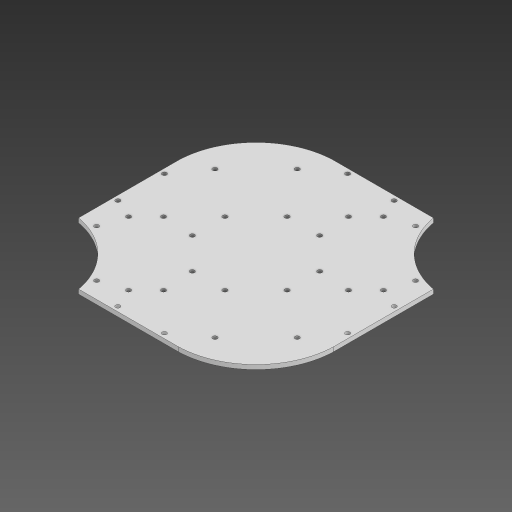
# Autodesk Inventor part: plat
Saved by Autodesk Inventor 2023 (Build 270158000, 158)
## iProperties
Created: 2025-06-24
Part Number: plat
Material: Типовые
Document SubType Name: Modeling
Designer: daa
Density: 1 g/cm^3
Appearance: По умолчанию
Author: daa
Autodesk Inventor part; units mm, degrees
ref_plane "YZ Plane" through (0, 0, 0) normal (1, 0, 0) x (0, 1, 0)
ref_plane "XZ Plane" through (0, 0, 0) normal (0, 1, 0) x (-1, 0, 0)
ref_plane "XY Plane" through (0, 0, 0) normal (0, 0, 1) x (1, 0, 0)
sketch "Эскиз1" plane through (0, 0, 0) normal (0, 1, 0) x (-1, 0, 0)
  line L0 (-79, -47.2724) -> (-79, 14.7276)
  line L1 (91.5447, -47.2724) -> (91.5447, 14.7276)
  line L2 (-79, -47.2724) -> (-93, -47.2724)
  line L3 (-79, 14.7276) -> (-93, 14.7276)
  line L4 (91.5447, -47.2724) -> (105.5447, -47.2724)
  line L5 (91.5447, 14.7276) -> (105.5447, 14.7276)
  line L6 (-24.7276, -101.5447) -> (37.2724, -101.5447)
  line L7 (-24.7276, 69) -> (37.2724, 69)
  line L8 (-24.7276, 69) -> (-24.7276, 83)
  line L9 (37.2724, 69) -> (37.2724, 83)
  line L10 (37.2724, -101.5447) -> (37.2724, -115.5447)
  line L11 (-24.7276, -101.5447) -> (-24.7276, -115.5447)
  arc A0 (-93, -47.2724) -> (-24.7276, -115.5447) centre (6.2724, -16.2724) ccw
  arc A1 (105.5447, 14.7276) -> (37.2724, 83) centre (6.2724, -16.2724) ccw
  arc A2 (-24.7276, 83) -> (-93, 14.7276) centre (6.2724, -16.2724) ccw
  arc A3 (37.2724, -115.5447) -> (105.5447, -47.2724) centre (6.2724, -16.2724) ccw
  dimension "d29" = 62
  dimension "d31" = 62
  dimension "d33" = 14
  dimension "d34" = 14
  dimension "d35" = 62
  dimension "d36" = 62
  dimension "d39" = 14
  dimension "d40" = 14
  dimension "d256" = 104
  dimension "d257" = 104
  dimension "d258" = 104
  dimension "d259" = 104
  dimension "d260" = 14
  dimension "d261" = 14
  dimension "d262" = 14
  dimension "d263" = 14
  dimension "d264" = 68.2724
  dimension "d265" = 68.2724
  dimension "d266" = 68.2724
  constraints: 24 end point, 8 point on circle, 4 centre point, 4 horizontal, 3 parallel, 3 vertical, 2 point on line, 1 concentric
  measures "d29" distance of L0.start L0.end
  measures "d31" distance of L1.start L1.end
  measures "d33" distance of L0.end L3.end
  measures "d34" distance of L1.end L5.end
  measures "d35" distance of L6.start L6.end
  measures "d36" distance of L7.start L7.end
  measures "d39" distance of L7.start L8.end
  measures "d40" distance of L6.start L11.end
  measures "d256" radius of A3
  measures "d257" radius of A0
  measures "d258" radius of A1
  measures "d259" radius of A2
  measures "d260" distance of L1.start L4.end
  measures "d261" distance of L6.end L10.end
  measures "d262" distance of L0.start L2.end
  measures "d263" distance of L7.end L9.end
  measures "d264" horizontal distance of L10.end L4.end
  measures "d265" horizontal distance of L2.end L11.end
  measures "d266" horizontal distance of L3.end A2.start
extrude "motor" add sketch "Эскиз1" along normal blind 3
sketch "Эскиз2" plane through (0, 3, 0) normal (0, 1, 0) x (1, 0, 0)
  arc A0 (24.7276, -83) -> (93, -14.7276) centre (-6.2724, 16.2724) ccw projected
  arc A1 (-37.2724, 115.5447) -> (-105.5447, 47.2724) centre (-6.2724, 16.2724) ccw projected
  circle A2 centre (-6.2724, 16.2724) radius 104
  line L0 (-6.2724, 16.2724) -> (-6.2724, -50.7276)
  arc A3 (-37.2724, 115.5447) -> (-105.5447, 47.2724) centre (-6.2724, 16.2724) ccw projected
  line L1 (-88.7917, -14.3063) -> (-40.8426, -62.2554)
  line L2 (-101.3809, -25.8032) -> (-48.3479, -78.8362)
  arc A4 (-105.5447, -14.7276) -> (-37.2724, -83) centre (-6.2724, 16.2724) ccw projected
  arc A5 (-48.3479, -78.8362) -> (-101.3809, -25.8032) centre (-98.035, -75.4903) ccw
  arc A6 (24.7276, -83) -> (93, -14.7276) centre (-6.2724, 16.2724) ccw projected
  line L3 (-79.8115, 89.8115) -> (67.2668, -57.2668)
  line L4 (24.3063, 98.7917) -> (72.2554, 50.8426)
  line L5 (35.8032, 111.3809) -> (88.8362, 58.3479)
  arc A7 (93, 47.2724) -> (24.7276, 115.5447) centre (-6.2724, 16.2724) ccw
  arc A8 (35.8032, 111.3809) -> (88.8362, 58.3479) centre (85.4903, 108.035) ccw
  line L6 (-91.5447, -14.7276) -> (-105.5447, -14.7276) projected
  arc A9 (-105.5447, -14.7276) -> (-101.3809, -25.8032) centre (-6.2724, 16.2724) ccw
  line L7 (-105.5447, -14.7276) -> (-80, -14.7276)
  point P0 (0, 0)
  point P1 (-6.2724, -50.7276)
  dimension "d181" = 208
  dimension "d190" = 67
  dimension "d205" = 75
  dimension "d207" = 17.0315
  dimension "d208" = 11.0756
  dimension "d209" = 104
  constraints: 14 end point, 10 point on circle, 7 symmetric about line, 5 centre point, 2 tangent, 1 point on line, 1 vertical, 2 other
  measures "d181" diameter of A2
  measures "d190" distance of L0.end L0.start
  measures "d205" distance of L2.start L2.end
  measures "d207" distance between parallel lines of L1 L2
  measures "d208" horizontal distance of A2.end L2.end
  measures "d209" radius of A9
extrude "ball" cut sketch "Эскиз2" against normal blind 3 contours A2 L2 | L2 A5 | L5 A2 | A8 L5
sketch "Эскиз3" plane through (0, 3, 0) normal (0, 1, 0) x (1, 0, 0)
  arc A0 (93, 47.2724) -> (24.7276, 115.5447) centre (-6.2724, 16.2724) ccw projected
  line L0 (-6.2724, 16.2724) -> (97.7276, 16.2724) construction
  line L1 (67.2668, 89.8115) -> (-62.5447, -40)
  circle A1 centre (70.5306, -44.2673) radius 1.5
  circle A2 centre (54.2672, -60.5308) radius 1.5
  circle A3 centre (41.3053, -71.6104) radius 1.5
  circle A4 centre (81.6104, -31.3053) radius 1.5
  arc A5 (24.7276, -83) -> (93, -14.7276) centre (-6.2724, 16.2724) ccw projected
  line L2 (-6.2724, 16.2724) -> (97.7276, 16.2724) construction
  line L3 (-79.8115, 89.8115) -> (67.2668, -57.2668)
  line L4 (-91.5447, 47.2724) -> (-91.5447, -14.7276) projected
  line L5 (-91.5447, 16.2724) -> (79, 16.2724)
  line L6 (24.7276, 101.5447) -> (-37.2724, 101.5447) projected
  line L7 (-6.2724, 101.5447) -> (-6.2724, -69)
  line L8 (-6.2724, 101.5447) -> (-6.2724, -69)
  line L9 (-91.5447, 47.2724) -> (-91.5447, -14.7276) projected
  arc A6 (24.7276, -83) -> (93, -14.7276) centre (-6.2724, 16.2724) ccw projected
  circle A7 centre (-66.812, 93.0753) radius 1.5
  circle A8 centre (-83.0755, 76.8119) radius 1.5
  circle A9 centre (-94.1551, 63.85) radius 1.5
  circle A10 centre (-53.85, 104.1551) radius 1.5
  point P0 (0, 0)
  point P1 (67.2668, -57.2668)
  point P2 (67.2668, -57.2668)
  point P3 (-105.5447, 47.2724)
  point P4 (-79.8115, 89.8115)
  point P5 (-79.8115, 89.8115)
  point P6 (-79.8115, 89.8115)
  dimension "d65" = 3
  dimension "d66" = 3
  dimension "d67" = 3
  dimension "d68" = 3
  dimension "d69" = 23
  dimension "d71" = 57
  dimension "d74" = -12.962
  dimension "d78" = 25.9614
  constraints: 14 end point, 8 centre point, 8 symmetric about line, 4 point on circle, 3 midpoint, 2 horizontal, 2 vertical, 1 point on line, 4 other
  measures "d65" diameter of A1
  measures "d66" diameter of A2
  measures "d67" diameter of A3
  measures "d68" diameter of A4
  measures "d69" distance of A2.centre A1.centre
  measures "d71" distance of A3.centre A4.centre
  measures "d74" vertical distance of A1.centre A4.centre
  measures "d78" vertical distance of A4.centre point (67.267, -57.267)
extrude "hand_mount" cut sketch "Эскиз3" against normal blind 10
sketch "Эскиз5" plane through (0, 3, 0) normal (0, 1, 0) x (1, 0, 0)
  circle A0 centre (29.7645, -47.992) radius 1.5
  circle A1 centre (58.0485, -19.7074) radius 1.5
  circle A2 centre (-6.2982, 16.355) radius 104
  arc A3 (-105.5447, -14.7276) -> (-99.04, -30.7083) centre (-6.2982, 16.355) ccw projected
  line L0 (-6.2982, 16.355) -> (97.7018, 16.355) construction
  line L1 (67.2409, 89.8941) -> (-79.8373, -57.1841)
  circle A4 centre (-70.6452, 52.4178) radius 1.5
  circle A5 centre (-42.3607, 80.7017) radius 1.5
  circle A6 centre (-44.9008, -54.7745) radius 1.5
  line L2 (-46.7704, -39.7817) -> (-62, -24)
  arc A7 (-53.253, -76.4953) -> (-99.04, -30.7083) centre (-88.8109, -66.2662) ccw projected
  line L3 (-62.7022, -40.049) -> (-61.1643, -38.511)
  line L4 (-61.1643, -38.511) -> (-44.8852, -38.511) construction
  line L5 (-61.1643, -38.511) -> (-44.9008, -54.7745)
  circle A8 centre (-77.4277, -22.2476) radius 1.5
  arc A9 (24.7276, -83) -> (93, -14.7276) centre (-6.2724, 16.2724) ccw projected
  line L6 (-6.2982, 16.355) -> (97.7785, 16.355) construction
  line L7 (67.2952, -57.2383) -> (-79.783, 89.8399)
  arc A10 (-37.2724, 115.5447) -> (-105.5447, 47.2724) centre (-6.2724, 16.2724) ccw projected
  circle A11 centre (64.8313, 54.9576) radius 1.5
  circle A12 centre (32.3044, 87.4845) radius 1.5
  point P0 (0, 0)
  dimension "d119" = 208
  dimension "d116" = 3
  dimension "d117" = 3
  dimension "d118" = 40
  dimension "d121" = 64.347
  dimension "d126" = 3
  dimension "d130" = 2.175
  dimension "d133" = 23
  constraints: 16 end point, 8 centre point, 5 symmetric about line, 4 point on circle, 3 horizontal, 2 point on line, 1 coincident, 9 other
  measures "d116" diameter of A0
  measures "d117" diameter of A1
  measures "d118" distance of A1.centre A0.centre
  measures "d121" vertical distance of L0.start A0.centre
  measures "d126" diameter of A6
  measures "d130" distance of L3.start L3.end
  measures "d133" distance of L3.end L5.end
extrude "Выдавливание5" cut sketch "Эскиз5" against normal blind 10 contours A0 | A1 | A4 | A5 | A6 | A8 | A11 | A12
sketch "Эскиз6" plane through (0, 3, 0) normal (0, 1, 0) x (1, 0, 0)
  circle A0 centre (-22.2724, 95.2947) radius 1.5
  circle A1 centre (9.7276, 95.2947) radius 1.5
  line L0 (24.7276, 115.5447) -> (24.7276, 101.5447) projected
  line L1 (24.7276, 101.5447) -> (-37.2724, 101.5447) projected
  circle A2 centre (-22.2724, -62.75) radius 1.5
  circle A3 centre (9.7276, -62.75) radius 1.5
  circle A4 centre (-85.2947, 32.2724) radius 1.5
  circle A5 centre (-85.2947, 0.2724) radius 1.5
  circle A6 centre (72.75, 32.2724) radius 1.5
  circle A7 centre (72.75, 0.2724) radius 1.5
  point P0 (0, 0)
  point P1 (24.7276, -69)
  point P2 (-37.2724, -69)
  point P3 (-91.5447, -14.7276)
  point P4 (-91.5447, 47.2724)
  point P5 (79, 47.2724)
  point P6 (79, -14.7276)
  dimension "d135" = 3
  dimension "d136" = 3
  dimension "d137" = 32
  dimension "d138" = 15
  dimension "d139" = 6.25
  dimension "d140" = 3
  dimension "d141" = 3
  dimension "d142" = 6.25
  dimension "d143" = 32
  dimension "d144" = 15
  dimension "d145" = 6.25
  dimension "d146" = 6.25
  dimension "d147" = 3
  dimension "d148" = 3
  dimension "d149" = 32
  dimension "d150" = 15
  dimension "d151" = 6.25
  dimension "d152" = 6.25
  dimension "d153" = 3
  dimension "d154" = 3
  dimension "d155" = 32
  dimension "d156" = 15
  dimension "d157" = 6.25
  dimension "d158" = 6.25
  constraints: 8 centre point
  measures "d135" diameter of A0
  measures "d136" diameter of A1
  measures "d137" distance of A1.centre A0.centre
  measures "d138" distance from line of L0 A1.centre
  measures "d139" distance from line of L1 A1.centre
  measures "d140" diameter of A2
  measures "d141" diameter of A3
  measures "d142" distance from line of L1 A0.centre
  measures "d143" distance of A2.centre A3.centre
  measures "d144" horizontal distance of point (24.728, -69) A3.centre
  measures "d145" vertical distance of point (24.728, -69) A3.centre
  measures "d146" vertical distance of point (-37.272, -69) A2.centre
  measures "d147" diameter of A4
  measures "d148" diameter of A5
  measures "d149" distance of A5.centre A4.centre
  measures "d150" vertical distance of A5.centre point (-91.545, -14.728)
  measures "d151" horizontal distance of A5.centre point (-91.545, -14.728)
  measures "d152" horizontal distance of A4.centre point (-91.545, 47.272)
  measures "d153" diameter of A6
  measures "d154" diameter of A7
  measures "d155" distance of A7.centre A6.centre
  measures "d156" vertical distance of point (79, 47.272) A6.centre
  measures "d157" horizontal distance of point (79, -14.728) A7.centre
  measures "d158" horizontal distance of point (79, 47.272) A6.centre
extrude "Выдавливание6" cut sketch "Эскиз6" against normal blind 10
fillet "Сопряжение1" radius 2 20 edges at (88.8362, 1.5, -58.3479) (35.8032, 1.5, -111.3809) (93, 1.5, -47.2724) (24.7276, 1.5, -115.5447) (24.7276, 1.5, -101.5447) (-37.2724, 1.5, -101.5447) (-37.2724, 1.5, -115.5447) (-105.5447, 1.5, -47.2724) (-91.5447, 1.5, -47.2724) (-91.5447, 1.5, 14.7276) (-105.5447, 1.5, 14.7276) (-48.3479, 1.5, 78.8362) (-101.3809, 1.5, 25.8032) (-37.2724, 1.5, 83) (-37.2724, 1.5, 69) (24.7276, 1.5, 69) (24.7276, 1.5, 83) (93, 1.5, 14.7276) (79, 1.5, 14.7276) (79, 1.5, -47.2724)
fillet_without_effect "Сопряжение4"
sketch "Эскиз8" plane through (0, 3, 0) normal (0, 1, 0) x (1, 0, 0)
  circle A0 centre (-75.6509, 84.2365) radius 1.6
  circle A1 centre (62.8514, -51.4283) radius 1.6
  circle A2 centre (-83.0755, 76.8119) radius 1.5
  circle A3 centre (-83.0755, 76.8119) radius 1.5 projected
  line L0 (-83.0755, 76.8119) -> (-75.6509, 84.2365)
  line L1 (-83.0755, 76.8119) -> (-72.5755, 76.8119) construction
  circle A4 centre (54.2672, -60.5308) radius 1.5
  circle A5 centre (54.2672, -60.5308) radius 1.5 projected
  line L2 (54.2672, -60.5308) -> (67.7672, -60.5308) construction
  circle A6 centre (70.5306, -44.2673) radius 1.5
  circle A7 centre (70.5306, -44.2673) radius 1.5 projected
  line L3 (70.5306, -44.2673) -> (62.8514, -51.4283)
  line L4 (70.5306, -44.2673) -> (81.0306, -44.2673) construction
  point P0 (0, 0)
  dimension "d211" = 3.2
  dimension "d212" = 3.2
  dimension "d213" = 3
  dimension "d214" = 10.5
  dimension "d215" = 45
  dimension "d216" = 3
  dimension "d221" = 3
  dimension "d222" = 10.5
  dimension "d223" = 137
  constraints: 10 end point, 5 centre point, 3 concentric, 3 horizontal, 2 coincident, 2 equal length
  measures "d211" diameter of A0
  measures "d212" diameter of A1
  measures "d213" diameter of A2
  measures "d214" distance of L0.start L0.end
  measures "d215" angle of L1 L0
  measures "d216" diameter of A4
  measures "d221" diameter of A6
  measures "d222" distance of L3.start L3.end
  measures "d223" angle of L3 L4
extrude "Выдавливание7" cut sketch "Эскиз8" against normal blind 10 contours A0 | A1
sketch "Эскиз9" plane through (0, 3, 0) normal (0, 1, 0) x (1, 0, 0)
  line L0 (-38.87, 27.5154) -> (-17.5154, 48.87)
  line L1 (-17.5154, 48.87) -> (26.3253, 5.0294)
  line L2 (26.3253, 5.0294) -> (4.9706, -16.3253)
  line L3 (4.9706, -16.3253) -> (-38.87, 27.5154)
  circle A0 centre (-6.2724, 16.2724) radius 104
  arc A1 (-39.9194, 114.679) -> (-104.679, 49.9194) centre (-6.2724, 16.2724) ccw projected
  circle A2 centre (-17.5154, 48.87) radius 1.5
  circle A3 centre (-38.87, 27.5154) radius 1.5
  circle A4 centre (4.9706, -16.3253) radius 1.5
  circle A5 centre (26.3253, 5.0294) radius 1.5
  point P0 (0, 0)
  dimension "d224" = 30.2
  dimension "d225" = 62
  dimension "d226" = 208
  dimension "d227" = 15.1
  dimension "d229" = 31
  dimension "d230" = 3
  dimension "d231" = 3
  dimension "d232" = 3
  dimension "d233" = 3
  constraints: 8 end point, 5 centre point, 4 coincident, 2 parallel, 1 concentric, 1 perpendicular
  measures "d224" distance of L1.end L2.end
  measures "d225" distance of L0.end L1.end
  measures "d226" diameter of A0
  measures "d227" distance from line of L1 A0.centre
  measures "d229" distance from line of L2 A0.centre
  measures "d230" diameter of A2
  measures "d231" diameter of A3
  measures "d232" diameter of A4
  measures "d233" diameter of A5
extrude "Выдавливание8" cut sketch "Эскиз9" against normal blind 10 contours L3 A3 L0 | L0 A3 L3 | A2 L1 L0 | L0 L1 A2 | A4 L2 L3 | L3 L2 A4 | A5 L2 L1 | L1 L2 A5
sketch "Эскиз10" plane through (0, 3, 0) normal (0, 1, 0) x (1, 0, 0)
  circle A0 centre (-6.2724, 16.2719) radius 104.0005
  arc A1 (-39.9194, 114.679) -> (-104.679, 49.9194) centre (-6.2724, 16.2724) ccw projected
  line L0 (-60.0125, 6.3729) -> (-72.0333, -5.648)
  line L1 (-72.0333, -5.648) -> (-28.1927, -49.4886)
  line L2 (-28.1927, -49.4886) -> (-16.1718, -37.4678)
  line L3 (-16.1718, -37.4678) -> (-60.0125, 6.3729)
  circle A2 centre (-60.0125, 6.3729) radius 1.5
  circle A3 centre (-72.0333, -5.648) radius 1.5
  circle A4 centre (-16.1718, -37.4678) radius 1.5
  circle A5 centre (-28.1927, -49.4886) radius 1.5
  line L4 (-6.2724, 16.2724) -> (67.2668, -57.2668)
  arc A6 (27.3747, -82.1343) -> (92.1343, -17.3747) centre (-6.2724, 16.2724) ccw projected
  line L5 (-6.2724, 16.2724) -> (97.7276, 16.2724) construction
  line L6 (67.2668, -57.2668) -> (-79.8115, 89.8115)
  line L7 (3.6271, 70.0125) -> (15.648, 82.0333)
  line L8 (15.648, 82.0333) -> (59.4886, 38.1927)
  line L9 (59.4886, 38.1927) -> (47.4678, 26.1718)
  line L10 (47.4678, 26.1718) -> (3.6271, 70.0125)
  circle A7 centre (3.6271, 70.0125) radius 1.5
  circle A8 centre (15.648, 82.0333) radius 1.5
  circle A9 centre (47.4678, 26.1718) radius 1.5
  circle A10 centre (59.4886, 38.1927) radius 1.5
  point P0 (0, 0)
  point P1 (10, 10)
  point P2 (-6.2719, 16.2724)
  dimension "d248" = 17
  dimension "d249" = 62
  dimension "d250" = 9.899
  dimension "d251" = 45
  dimension "d252" = 3
  dimension "d253" = 3
  dimension "d254" = 3
  dimension "d255" = 3
  dimension "d282" = 45
  constraints: 22 end point, 10 symmetric about line, 9 centre point, 8 coincident, 2 parallel, 2 point on circle, 1 equal length, 1 horizontal, 1 perpendicular, 1 point on line, 1 tangent, 4 other
  measures "d248" distance of L2.end L1.end
  measures "d249" distance of L1.end L0.end
  measures "d250" vertical distance of L0.start A0.centre
  measures "d251" distance from line of L3 L4.start
  measures "d252" diameter of A2
  measures "d253" diameter of A3
  measures "d254" diameter of A4
  measures "d255" diameter of A5
  measures "d282" angle of L4 L5
extrude "Выдавливание9" cut sketch "Эскиз10" against normal blind 10 contours L3 A2 L0 | L0 A2 L3 | A3 L1 L0 | L0 L1 A3 | A4 L2 L3 | L3 L2 A4 | A5 L2 L1 | L1 L2 A5 | L10 A7 L7 | L7 A7 L10 | A8 L8 L7 | L7 L8 A8 | A9 L9 L10 | L10 L9 A9 | A10 L9 L8 | L8 L9 A10
sketch "Эскиз14" plane through (0, 3, 0) normal (0, 1, 0) x (1, 0, 0)
  line L0 (-38.8696, 5.0294) -> (4.971, 48.87)
  line L1 (4.971, 48.87) -> (26.3256, 27.5154)
  line L2 (26.3256, 27.5154) -> (-17.515, -16.3253)
  line L3 (-17.515, -16.3253) -> (-38.8696, 5.0294)
  circle A0 centre (47.4678, 26.1718) radius 1.5 projected
  circle A1 centre (-28.1927, -49.4886) radius 1.5 projected
  circle A2 centre (-72.0333, -5.648) radius 1.5 projected
  circle A3 centre (15.648, 82.0333) radius 1.5 projected
  circle A4 centre (59.4886, 38.1927) radius 1.5 projected
  circle A5 centre (-16.1718, -37.4678) radius 1.5 projected
  circle A6 centre (-60.0125, 6.3729) radius 1.5 projected
  circle A7 centre (3.6271, 70.0125) radius 1.5 projected
  circle A8 centre (4.9706, -16.3253) radius 1.5 projected
  circle A9 centre (-17.5154, 48.87) radius 1.5 projected
  circle A10 centre (26.3253, 5.0294) radius 1.5 projected
  circle A11 centre (-38.87, 27.5154) radius 1.5 projected
  circle A12 centre (62.8514, -51.4283) radius 1.6 projected
  circle A13 centre (-75.6509, 84.2365) radius 1.6 projected
  arc A14 (89.3952, 57.061) -> (87.4757, 58.275) centre (87.5555, 56.2766) ccw projected
  arc A15 (35.7303, 110.0204) -> (87.4757, 58.275) centre (85.4903, 108.035) ccw projected
  arc A16 (35.7303, 110.0204) -> (34.5163, 111.9399) centre (33.7319, 110.1002) ccw projected
  arc A17 (34.5163, 111.9399) -> (27.3747, 114.679) centre (-6.2724, 16.2724) ccw projected
  arc A18 (27.3747, 114.679) -> (24.7276, 112.7866) centre (26.7276, 112.7866) ccw projected
  line L4 (24.7276, 112.7866) -> (24.7276, 103.5447) projected
  arc A19 (22.7276, 101.5447) -> (24.7276, 103.5447) centre (22.7276, 103.5447) ccw projected
  line L5 (22.7276, 101.5447) -> (-35.2724, 101.5447) projected
  arc A20 (-37.2724, 103.5447) -> (-35.2724, 101.5447) centre (-35.2724, 103.5447) ccw projected
  line L6 (-37.2724, 103.5447) -> (-37.2724, 112.7866) projected
  arc A21 (-37.2724, 112.7866) -> (-39.9194, 114.679) centre (-39.2724, 112.7866) ccw projected
  arc A22 (-39.9194, 114.679) -> (-104.679, 49.9194) centre (-6.2724, 16.2724) ccw projected
  arc A23 (-104.679, 49.9194) -> (-102.7866, 47.2724) centre (-102.7866, 49.2724) ccw projected
  line L7 (-102.7866, 47.2724) -> (-93.5447, 47.2724) projected
  arc A24 (-91.5447, 45.2724) -> (-93.5447, 47.2724) centre (-93.5447, 45.2724) ccw projected
  line L8 (-91.5447, 45.2724) -> (-91.5447, -12.7276) projected
  arc A25 (-93.5447, -14.7276) -> (-91.5447, -12.7276) centre (-93.5447, -12.7276) ccw projected
  line L9 (-93.5447, -14.7276) -> (-102.7866, -14.7276) projected
  arc A26 (-102.7866, -14.7276) -> (-104.679, -17.3747) centre (-102.7866, -16.7276) ccw projected
  arc A27 (-104.679, -17.3747) -> (-101.9399, -24.5163) centre (-6.2724, 16.2724) ccw projected
  arc A28 (-101.9399, -24.5163) -> (-100.0204, -25.7303) centre (-100.1002, -23.7319) ccw projected
  arc A29 (-48.275, -77.4757) -> (-100.0204, -25.7303) centre (-98.035, -75.4903) ccw projected
  arc A30 (-48.275, -77.4757) -> (-47.061, -79.3952) centre (-46.2766, -77.5555) ccw projected
  arc A31 (-47.061, -79.3952) -> (-39.9194, -82.1343) centre (-6.2724, 16.2724) ccw projected
  arc A32 (-39.9194, -82.1343) -> (-37.2724, -80.2419) centre (-39.2724, -80.2419) ccw projected
  line L10 (-37.2724, -80.2419) -> (-37.2724, -71) projected
  arc A33 (-35.2724, -69) -> (-37.2724, -71) centre (-35.2724, -71) ccw projected
  line L11 (-35.2724, -69) -> (22.7276, -69) projected
  arc A34 (24.7276, -71) -> (22.7276, -69) centre (22.7276, -71) ccw projected
  line L12 (24.7276, -71) -> (24.7276, -80.2419) projected
  arc A35 (24.7276, -80.2419) -> (27.3747, -82.1343) centre (26.7276, -80.2419) ccw projected
  arc A36 (27.3747, -82.1343) -> (92.1343, -17.3747) centre (-6.2724, 16.2724) ccw projected
  arc A37 (92.1343, -17.3747) -> (90.2419, -14.7276) centre (90.2419, -16.7276) ccw projected
  line L13 (90.2419, -14.7276) -> (81, -14.7276) projected
  arc A38 (79, -12.7276) -> (81, -14.7276) centre (81, -12.7276) ccw projected
  line L14 (79, -12.7276) -> (79, 45.2724) projected
  arc A39 (81, 47.2724) -> (79, 45.2724) centre (81, 45.2724) ccw projected
  line L15 (81, 47.2724) -> (90.2419, 47.2724) projected
  arc A40 (90.2419, 47.2724) -> (92.1343, 49.9194) centre (90.2419, 49.2724) ccw projected
  arc A41 (92.1343, 49.9194) -> (89.3952, 57.061) centre (-6.2724, 16.2724) ccw projected
  circle A42 centre (-94.1551, 63.85) radius 1.5 projected
  circle A43 centre (41.3053, -71.6104) radius 1.5 projected
  circle A44 centre (81.6104, -31.3053) radius 1.5 projected
  circle A45 centre (-53.85, 104.1551) radius 1.5 projected
  circle A46 centre (-83.0755, 76.8119) radius 1.5 projected
  circle A47 centre (54.2672, -60.5308) radius 1.5 projected
  circle A48 centre (70.5306, -44.2673) radius 1.5 projected
  circle A49 centre (-66.812, 93.0753) radius 1.5 projected
  circle A50 centre (-44.9008, -54.7745) radius 1.5 projected
  circle A51 centre (29.7645, -47.992) radius 1.5 projected
  circle A52 centre (-42.3607, 80.7017) radius 1.5 projected
  circle A53 centre (32.3044, 87.4845) radius 1.5 projected
  circle A54 centre (-77.4277, -22.2476) radius 1.5 projected
  circle A55 centre (58.0485, -19.7074) radius 1.5 projected
  circle A56 centre (-70.6452, 52.4178) radius 1.5 projected
  circle A57 centre (64.8313, 54.9576) radius 1.5 projected
  circle A58 centre (-85.2947, 0.2724) radius 1.5 projected
  circle A59 centre (72.75, 0.2724) radius 1.5 projected
  circle A60 centre (-22.2724, 95.2947) radius 1.5 projected
  circle A61 centre (9.7276, -62.75) radius 1.5 projected
  circle A62 centre (-85.2947, 32.2724) radius 1.5 projected
  circle A63 centre (72.75, 32.2724) radius 1.5 projected
  circle A64 centre (9.7276, 95.2947) radius 1.5 projected
  circle A65 centre (-22.2724, -62.75) radius 1.5 projected
  circle A66 centre (-38.8696, 5.0294) radius 1.5
  circle A67 centre (-17.515, -16.3253) radius 1.5
  circle A68 centre (4.971, 48.87) radius 1.5
  circle A69 centre (26.3256, 27.5154) radius 1.5
  point P0 (0, 0)
  dimension "d283" = 30.2
  dimension "d284" = 62
  dimension "d285" = 32.598
  dimension "d286" = 32.5976
  dimension "d287" = 3
  dimension "d288" = 3
  dimension "d289" = 3
  dimension "d290" = 3
  constraints: 8 end point, 4 centre point, 4 coincident, 2 parallel, 1 perpendicular
  measures "d283" distance of L0.end L1.end
  measures "d284" distance of L1.end L2.end
  measures "d285" horizontal distance of L1.end A22.centre
  measures "d286" vertical distance of L0.end A31.centre
  measures "d287" diameter of A66
  measures "d288" diameter of A67
  measures "d289" diameter of A68
  measures "d290" diameter of A69
sketch "Эскиз13" plane through (0, 3, 0) normal (0, 1, 0) x (1, 0, 0)
  circle A0 centre (-28.1927, -49.4886) radius 1.5 projected
  circle A1 centre (-72.0333, -5.648) radius 1.5 projected
  circle A2 centre (-16.1718, -37.4678) radius 1.5 projected
  circle A3 centre (-60.0125, 6.3729) radius 1.5 projected
  circle A4 centre (4.9706, -16.3253) radius 1.5 projected
  circle A5 centre (-17.5154, 48.87) radius 1.5 projected
  circle A6 centre (26.3253, 5.0294) radius 1.5 projected
  circle A7 centre (-38.87, 27.5154) radius 1.5 projected
  circle A8 centre (62.8514, -51.4283) radius 1.6 projected
  circle A9 centre (-75.6509, 84.2365) radius 1.6 projected
  arc A10 (89.3952, 57.061) -> (87.4757, 58.275) centre (87.5555, 56.2766) ccw projected
  arc A11 (35.7303, 110.0204) -> (87.4757, 58.275) centre (85.4903, 108.035) ccw projected
  arc A12 (35.7303, 110.0204) -> (34.5163, 111.9399) centre (33.7319, 110.1002) ccw projected
  arc A13 (34.5163, 111.9399) -> (27.3747, 114.679) centre (-6.2724, 16.2724) ccw projected
  arc A14 (27.3747, 114.679) -> (24.7276, 112.7866) centre (26.7276, 112.7866) ccw projected
  line L0 (24.7276, 112.7866) -> (24.7276, 103.5447) projected
  arc A15 (22.7276, 101.5447) -> (24.7276, 103.5447) centre (22.7276, 103.5447) ccw projected
  line L1 (22.7276, 101.5447) -> (-35.2724, 101.5447) projected
  arc A16 (-37.2724, 103.5447) -> (-35.2724, 101.5447) centre (-35.2724, 103.5447) ccw projected
  line L2 (-37.2724, 103.5447) -> (-37.2724, 112.7866) projected
  arc A17 (-37.2724, 112.7866) -> (-39.9194, 114.679) centre (-39.2724, 112.7866) ccw projected
  arc A18 (-39.9194, 114.679) -> (-104.679, 49.9194) centre (-6.2724, 16.2724) ccw projected
  arc A19 (-104.679, 49.9194) -> (-102.7866, 47.2724) centre (-102.7866, 49.2724) ccw projected
  line L3 (-102.7866, 47.2724) -> (-93.5447, 47.2724) projected
  arc A20 (-91.5447, 45.2724) -> (-93.5447, 47.2724) centre (-93.5447, 45.2724) ccw projected
  line L4 (-91.5447, 45.2724) -> (-91.5447, -12.7276) projected
  arc A21 (-93.5447, -14.7276) -> (-91.5447, -12.7276) centre (-93.5447, -12.7276) ccw projected
  line L5 (-93.5447, -14.7276) -> (-102.7866, -14.7276) projected
  arc A22 (-102.7866, -14.7276) -> (-104.679, -17.3747) centre (-102.7866, -16.7276) ccw projected
  arc A23 (-104.679, -17.3747) -> (-101.9399, -24.5163) centre (-6.2724, 16.2724) ccw projected
  arc A24 (-101.9399, -24.5163) -> (-100.0204, -25.7303) centre (-100.1002, -23.7319) ccw projected
  arc A25 (-48.275, -77.4757) -> (-100.0204, -25.7303) centre (-98.035, -75.4903) ccw projected
  arc A26 (-48.275, -77.4757) -> (-47.061, -79.3952) centre (-46.2766, -77.5555) ccw projected
  arc A27 (-47.061, -79.3952) -> (-39.9194, -82.1343) centre (-6.2724, 16.2724) ccw projected
  arc A28 (-39.9194, -82.1343) -> (-37.2724, -80.2419) centre (-39.2724, -80.2419) ccw projected
  line L6 (-37.2724, -80.2419) -> (-37.2724, -71) projected
  arc A29 (-35.2724, -69) -> (-37.2724, -71) centre (-35.2724, -71) ccw projected
  line L7 (-35.2724, -69) -> (22.7276, -69) projected
  arc A30 (24.7276, -71) -> (22.7276, -69) centre (22.7276, -71) ccw projected
  line L8 (24.7276, -71) -> (24.7276, -80.2419) projected
  arc A31 (24.7276, -80.2419) -> (27.3747, -82.1343) centre (26.7276, -80.2419) ccw projected
  arc A32 (27.3747, -82.1343) -> (92.1343, -17.3747) centre (-6.2724, 16.2724) ccw projected
  arc A33 (92.1343, -17.3747) -> (90.2419, -14.7276) centre (90.2419, -16.7276) ccw projected
  line L9 (90.2419, -14.7276) -> (81, -14.7276) projected
  arc A34 (79, -12.7276) -> (81, -14.7276) centre (81, -12.7276) ccw projected
  line L10 (79, -12.7276) -> (79, 45.2724) projected
  arc A35 (81, 47.2724) -> (79, 45.2724) centre (81, 45.2724) ccw projected
  line L11 (81, 47.2724) -> (90.2419, 47.2724) projected
  arc A36 (90.2419, 47.2724) -> (92.1343, 49.9194) centre (90.2419, 49.2724) ccw projected
  arc A37 (92.1343, 49.9194) -> (89.3952, 57.061) centre (-6.2724, 16.2724) ccw projected
  circle A38 centre (-94.1551, 63.85) radius 1.5 projected
  circle A39 centre (41.3053, -71.6104) radius 1.5 projected
  circle A40 centre (81.6104, -31.3053) radius 1.5 projected
  circle A41 centre (-53.85, 104.1551) radius 1.5 projected
  circle A42 centre (-83.0755, 76.8119) radius 1.5 projected
  circle A43 centre (54.2672, -60.5308) radius 1.5 projected
  circle A44 centre (70.5306, -44.2673) radius 1.5 projected
  circle A45 centre (-66.812, 93.0753) radius 1.5 projected
  circle A46 centre (-44.9008, -54.7745) radius 1.5 projected
  circle A47 centre (29.7645, -47.992) radius 1.5 projected
  circle A48 centre (-42.3607, 80.7017) radius 1.5 projected
  circle A49 centre (32.3044, 87.4845) radius 1.5 projected
  circle A50 centre (-77.4277, -22.2476) radius 1.5 projected
  circle A51 centre (58.0485, -19.7074) radius 1.5 projected
  circle A52 centre (-70.6452, 52.4178) radius 1.5 projected
  circle A53 centre (64.8313, 54.9576) radius 1.5 projected
  circle A54 centre (-85.2947, 0.2724) radius 1.5 projected
  circle A55 centre (72.75, 0.2724) radius 1.5 projected
  circle A56 centre (-22.2724, 95.2947) radius 1.5 projected
  circle A57 centre (9.7276, -62.75) radius 1.5 projected
  circle A58 centre (-85.2947, 32.2724) radius 1.5 projected
  circle A59 centre (72.75, 32.2724) radius 1.5 projected
  circle A60 centre (9.7276, 95.2947) radius 1.5 projected
  circle A61 centre (-22.2724, -62.75) radius 1.5 projected
  line L12 (-86.5447, -12.7276) -> (-86.5447, 45.2724)
  arc A62 (-86.5447, 45.2724) -> (-93.5447, 52.2724) centre (-93.5447, 45.2724) ccw
  line L13 (-93.5447, 52.2724) -> (-98.4949, 52.2724)
  arc A63 (-42.2724, 108.4949) -> (-98.4949, 52.2724) centre (-6.2724, 16.2724) ccw
  line L14 (-42.2724, 108.4949) -> (-42.2724, 103.5447)
  arc A64 (-42.2724, 103.5447) -> (-35.2724, 96.5447) centre (-35.2724, 103.5447) ccw
  line L15 (-35.2724, 96.5447) -> (22.7276, 96.5447)
  arc A65 (32.8155, 92.9235) -> (70.3788, 55.3602) centre (85.4903, 108.035) ccw
  line L16 (74, 45.2724) -> (74, -12.7276)
  arc A66 (74, -12.7276) -> (81, -19.7276) centre (81, -12.7276) ccw
  line L17 (81, -19.7276) -> (85.9502, -19.7276)
  arc A67 (29.7276, -75.9502) -> (85.9502, -19.7276) centre (-6.2724, 16.2724) ccw
  line L18 (29.7276, -75.9502) -> (29.7276, -71)
  arc A68 (29.7276, -71) -> (22.7276, -64) centre (22.7276, -71) ccw
  line L19 (22.7276, -64) -> (-35.2724, -64)
  arc A69 (-45.3602, -60.3788) -> (-82.9235, -22.8155) centre (-98.035, -75.4903) ccw
  line L20 (-35.2724, -69) -> (22.7276, -69) projected
  line L21 (-35.2724, -64) -> (-40.554, -64)
  line L22 (-86.5447, -12.7276) -> (-86.5447, -18.0093)
  line L23 (22.7276, 96.5447) -> (28.0093, 96.5447)
  line L24 (74, 45.2724) -> (74, 50.554)
  arc A70 (74, 50.554) -> (70.3788, 55.3602) centre (69, 50.554) ccw
  arc A71 (32.8155, 92.9235) -> (28.0093, 96.5447) centre (28.0093, 91.5447) ccw
  arc A72 (-86.5447, -18.0093) -> (-82.9235, -22.8155) centre (-81.5447, -18.0093) ccw
  arc A73 (-45.3602, -60.3788) -> (-40.554, -64) centre (-40.554, -59) ccw
  arc A74 (-82.3013, -18.0093) -> (-81.7533, -18.7365) centre (-81.5447, -18.0093) ccw
  line L25 (22.7276, -69) -> (-35.2724, -69)
  arc A75 (-35.2724, -66) -> (-40.2724, -71) centre (-35.2724, -71) ccw
  line L26 (-40.2724, -71) -> (-40.2724, -78.8329)
  arc A76 (-45.2543, -76.9017) -> (-40.2724, -78.8329) centre (-6.2724, 16.2724) ccw
  arc A77 (-45.2543, -76.9017) -> (-99.4464, -22.7096) centre (-98.035, -75.4903) ccw
  arc A78 (-101.3776, -17.7276) -> (-99.4464, -22.7096) centre (-6.2724, 16.2724) ccw
  line L27 (-101.3776, -17.7276) -> (-93.5447, -17.7276)
  arc A79 (-93.5447, -17.7276) -> (-88.5447, -12.7276) centre (-93.5447, -12.7276) ccw
  line L28 (-88.5447, -12.7276) -> (-88.5447, 45.2724)
  arc A80 (-88.5447, 45.2724) -> (-93.5447, 50.2724) centre (-93.5447, 45.2724) ccw
  line L29 (-93.5447, 50.2724) -> (-101.3776, 50.2724)
  arc A81 (-40.2724, 111.3776) -> (-101.3776, 50.2724) centre (-6.2724, 16.2724) ccw
  line L30 (-40.2724, 111.3776) -> (-40.2724, 103.5447)
  arc A82 (-40.2724, 103.5447) -> (-35.2724, 98.5447) centre (-35.2724, 103.5447) ccw
  line L31 (-35.2724, 98.5447) -> (22.7276, 98.5447)
  arc A83 (22.7276, 98.5447) -> (27.7276, 103.5447) centre (22.7276, 103.5447) ccw
  line L32 (27.7276, 103.5447) -> (27.7276, 111.3776)
  arc A84 (32.7096, 109.4464) -> (27.7276, 111.3776) centre (-6.2724, 16.2724) ccw
  arc A85 (32.7096, 109.4464) -> (86.9017, 55.2543) centre (85.4903, 108.035) ccw
  line L33 (76, 45.2724) -> (76, -12.7276)
  arc A86 (76, -12.7276) -> (81, -17.7276) centre (81, -12.7276) ccw
  line L34 (81, -17.7276) -> (88.8329, -17.7276)
  arc A87 (27.7276, -78.8329) -> (88.8329, -17.7276) centre (-6.2724, 16.2724) ccw
  line L35 (27.7276, -78.8329) -> (27.7276, -71)
  arc A88 (27.7276, -71) -> (22.7276, -66) centre (22.7276, -71) ccw
  line L36 (22.7276, -66) -> (-35.2724, -66)
  line L37 (76, 45.2724) -> (76, 56.0953)
  line L38 (-35.2724, -66) -> (-46.0953, -66)
  line L39 (22.7276, 98.5447) -> (33.5506, 98.5447)
  line L40 (-88.5447, -12.7276) -> (-88.5447, -23.5506)
  arc A89 (-35.2724, 98.5447) -> (-88.5447, 45.2724) centre (-33.571, 43.571) ccw
  arc A90 (22.7276, -66) -> (76, -12.7276) centre (21.0263, -11.0263) ccw
  point P0 (0, 0)
  point P1 (-44.4536, -64)
  point P2 (-86.5447, -21.9089)
  point P3 (31.9089, 96.5447)
  point P4 (74, 54.4536)
  point P5 (46.7411, 69.2858)
  point P6 (50.2767, 72.8214)
  point P7 (-93.8825, 62.375)
  point P8 (-92.771, 64.4282)
  point P9 (-84.575, 76.8504)
  point P10 (-83.4632, 78.2609)
  point P11 (-68.2611, 93.463)
  point P12 (-66.8506, 94.5748)
  point P13 (-54.4282, 102.771)
  point P14 (-52.375, 103.8825)
  point P15 (-23.1015, 96.5447)
  point P16 (-21.4432, 96.5447)
  point P17 (8.8985, 96.5447)
  point P18 (10.5568, 96.5447)
  point P19 (74, 33.1015)
  point P20 (74, 31.4432)
  point P21 (74, 1.1015)
  point P22 (74, -0.5568)
  point P23 (81.3378, -29.8303)
  point P24 (80.2263, -31.8835)
  point P25 (72.0301, -44.3059)
  point P26 (70.9183, -45.7164)
  point P27 (55.7162, -60.9185)
  point P28 (54.3057, -62.0303)
  point P29 (41.8835, -70.2263)
  point P30 (39.8303, -71.3378)
  point P31 (10.5568, -64)
  point P32 (8.8985, -64)
  point P33 (-21.4432, -64)
  point P34 (-23.1015, -64)
  point P35 (-86.5447, -0.5568)
  point P36 (-86.5447, 1.1015)
  point P37 (-86.5447, 31.4432)
  point P38 (-86.5447, 33.1015)
  point P39 (-95.5923, 63.4205)
  point P40 (-94.5811, 65.2883)
  point P41 (-55.2883, 104.5811)
  point P42 (-53.4205, 105.5923)
  point P43 (83.0476, -30.8758)
  point P44 (82.0364, -32.7436)
  point P45 (42.7436, -72.0364)
  point P46 (40.8758, -73.0476)
  dimension "d267" = 5
  dimension "d268" = 5
  dimension "d269" = 5
  dimension "d270" = 5
  dimension "d271" = 3.5355
  dimension "d276" = 3
  dimension "d279" = 55
  dimension "d281" = 55
  constraints: 68 point on circle, 56 end point, 29 centre point, 9 tangent, 4 point on line, 3 equal radius, 3 horizontal, 3 vertical, 2 equal length, 2 perpendicular, 34 other
  measures "d267" radial gap between concentric circles of A25 A69
  measures "d268" radius of A70
  measures "d269" distance between parallel lines of L19 L7
  measures "d270" distance between parallel lines of L1 L15
  measures "d271" horizontal distance of point (46.741, 69.286) point (50.277, 72.821)
  measures "d276" radial gap between concentric circles of A32 A87
  measures "d279" radius of A89
  measures "d281" radius of A90
extrude "Выдавливание11" cut sketch "Эскиз13" against normal blind 10 contours A37 A36 L11 A35 L10 A34 L9 A33 A32 A31 L8 A30 L7 A29 L6 A28 A27 A26 A25 A24 A23 A22 L5 A21 L4 A20 L3 A19 A18 A17 L2 A16 L1 A15 L0 A14 A13 A12 A11 A10 | A38 A63 A42 A45 A41 L14 A64 A89 A62 L13 | A38 A81 A41 A63 A45 A42 | A63 L13 A62 A89 A80 L29 A81 A38 | A81 L30 A82 A89 A64 L14 A63 A41 | L40 A77 A78 L27 A79 | A83 L32 A84 A85 L39 | L38 A75 L26 A76 A77 | A90 A68 L18 A67 A39 A87 L35 A88 | A90 A66 L17 A67 A40 A44 A43 A39 L18 A68 | A86 L34 A87 A40 A67 L17 A66 A90 | A39 A67 A43 A44 A40 A87
extrude "Выдавливание12" cut sketch "Эскиз14" against normal blind 10 contours L3 A66 L0 | L0 A66 L3 | A68 L1 L0 | L0 L1 A68 | A67 L2 L3 | L3 L2 A67 | A69 L2 L1 | L1 L2 A69
